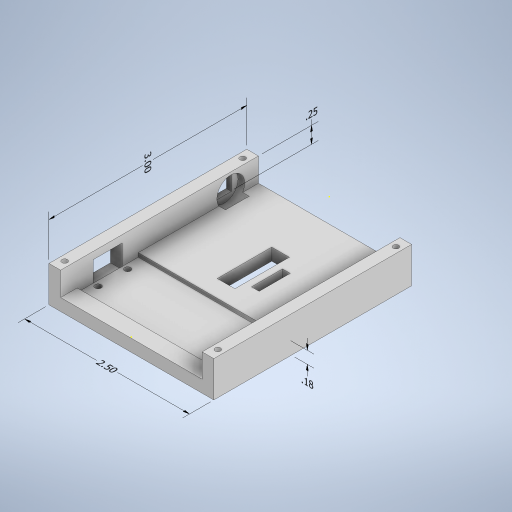
# Autodesk Inventor part: Scanner_Test_Top
Saved by Autodesk Inventor 2024 (Build 280153000, 153)
## iProperties
Created: 2022-09-22
Part Number: Scanner_Test_Top
Material: Generic
Document SubType Name: Modeling
Designer: Vking
Density: 1 g/cm^3
Appearance: Default
Author: Vking
Autodesk Inventor part; units mm, degrees
ref_plane "YZ Plane" through (0, 0, 0) normal (1, 0, 0) x (0, 1, 0)
ref_plane "XZ Plane" through (0, 0, 0) normal (0, 1, 0) x (-1, 0, 0)
ref_plane "XY Plane" through (0, 0, 0) normal (0, 0, 1) x (1, 0, 0)
sketch "Sketch1" plane through (0, 0, 0) normal (0, 0, 1) x (1, 0, 0)
  line L0 (-31.75, 5.08) -> (31.75, 5.08)
  line L1 (31.75, 5.08) -> (31.75, -5.08)
  line L2 (31.75, -5.08) -> (-31.75, -5.08)
  line L3 (-31.75, -5.08) -> (-31.75, 5.08)
  point P0 (0, 0)
  dimension "d0" = 63.5
  dimension "d3" = 31.75
  dimension "d4" = 10.16
  dimension "d17" = 5.08
  constraints: 8 end point, 2 parallel, 1 horizontal, 1 perpendicular
  measures "d0" distance of L0.start L0.end
  measures "d3" distance from line of L3 point (0, 0)
  measures "d4" distance of L0.end L1.end
  measures "d17" distance from line of point (0, 0) L2
extrude "Extrusion1" add sketch "Sketch1" along normal blind 76.2
sketch "Sketch3" plane through (0, 0, 76.2) normal (0, 0, 1) x (1, 0, 0)
  line L0 (-27.25, 0.3875) -> (27.25, 0.3875)
  line L1 (27.25, 0.3875) -> (27.25, -0.3745)
  line L2 (27.25, -0.3745) -> (-27.25, -0.3745)
  line L3 (-27.25, -0.3745) -> (-27.25, 0.3875)
  line L4 (-31.75, 5.08) -> (-31.75, -5.08) projected
  point P0 (0, 0)
  point P1 (-27.25, 0.0065)
  dimension "d6" = 0.762
  dimension "d7" = 54.5
  dimension "d8" = 4.5
  constraints: 8 end point, 2 parallel, 1 horizontal, 1 midpoint, 1 perpendicular
  measures "d6" distance between parallel lines of L2 L0
  measures "d7" distance of L0.start L0.end
  measures "d8" distance from line of L4 point (-27.25, 0.006)
extrude "Extrusion2" cut sketch "Sketch3" against normal blind 85.1
sketch "Sketch8" plane through (0, 0, 76.2) normal (0, 0, 1) x (1, 0, 0)
  line L0 (-31.75, -5.08) -> (31.75, -5.08) projected
  line L1 (31.75, -5.08) -> (31.75, 5.08) projected
  line L2 (-31.75, -5.08) -> (31.75, -5.08)
  line L3 (31.75, -5.08) -> (31.75, 0.3875)
  line L4 (31.75, 0.3875) -> (-31.75, 0.3875)
  line L5 (27.25, 0.3875) -> (27.25, -0.3745) projected
  line L6 (27.25, -0.3745) -> (-27.25, -0.3745) projected
  line L7 (-27.25, -0.3745) -> (-27.25, 0.3875) projected
  line L8 (-27.25, 0.3875) -> (27.25, 0.3875) projected
  line L9 (-31.75, -5.08) -> (31.75, -5.08) projected
  line L10 (31.75, -5.08) -> (31.75, 5.08) projected
  line L11 (31.75, 5.08) -> (-31.75, 5.08) projected
  line L12 (-31.75, 5.08) -> (-31.75, -5.08) projected
  line L13 (-27.25, 0.3875) -> (-27.25, -0.3745) projected
  line L14 (-27.25, 0.3875) -> (27.25, 0.3875)
  line L15 (27.25, 0.3875) -> (27.25, -5.08)
  line L16 (27.25, -5.08) -> (-27.25, -5.08)
  line L17 (-27.25, -5.08) -> (-27.25, 0.3875)
  point P0 (0, 0)
  dimension "d30" = 0
  constraints: 14 end point, 3 parallel, 2 horizontal, 2 perpendicular, 2 point on line
  measures "d30" distance between parallel lines of L8 L4
sketch "Sketch9" plane through (-31.75, 5.08, 0) normal (0, 1, 0) x (1, 0, 0)
  line L0 (28.35, -18.7333) -> (35.15, -18.7333)
  line L1 (35.15, -18.7333) -> (35.15, -39.7333)
  line L2 (35.15, -39.7333) -> (28.35, -39.7333)
  line L3 (28.35, -39.7333) -> (28.35, -18.7333)
  line L4 (0, 0) -> (0, -76.2) projected
  line L5 (63.5, 0) -> (0, 0) projected
  point P0 (31.75, 0)
  point P1 (0, -38.1)
  dimension "d31" = 21
  dimension "d32" = 6.8
  dimension "d33" = 28.35
  dimension "d34" = 18.7333
  constraints: 8 end point, 2 parallel, 1 horizontal, 1 midpoint, 1 perpendicular
  measures "d31" distance of L0.end L1.end
  measures "d32" distance of L1.end L2.end
  measures "d33" distance from line of point (0, -38.1) L3
  measures "d34" distance between parallel lines of L0 L5
extrude "Extrusion6" cut sketch "Sketch8" against normal blind 76.2 contours L17 L6 L15 L0
sketch "Sketch11" plane through (0, 0, 76.2) normal (0, 0, 1) x (1, 0, 0)
  point P0 (0, 0)
sketch "Sketch12" plane through (-31.75, -5.08, 0) normal (0, -1, 0) x (1, 0, 0)
  line L0 (4.5, 0) -> (4.5, 76.2) projected
  line L1 (0, 76.2) -> (4.5, 76.2) projected
  line L2 (0, 0) -> (0, 76.2) projected
  line L3 (0, 0) -> (4.5, 0) projected
  line L4 (59, 76.2) -> (59, 0) projected
  line L5 (59, 0) -> (63.5, 0) projected
  line L6 (63.5, 0) -> (63.5, 76.2) projected
  line L7 (59, 76.2) -> (63.5, 76.2) projected
  point P0 (31.75, 0)
extrude "Extrusion7" add sketch "Sketch12" along normal blind 3.641
extrude "Extrusion8" cut sketch "Sketch9" against normal blind 19.5
sketch "Sketch13" plane through (-31.75, -8.721, 0) normal (0, -1, 0) x (1, 0, 0)
  point P0 (31.75, 0)
sketch "Sketch14" plane through (27.25, 0.3875, 0) normal (-1, 0, 0) x (0, 0, 1)
  circle A0 centre (10.668, -2.7585) radius 5.334
  line L0 (76.2, 0) -> (0, 0) projected
  line L1 (76.2, -9.1085) -> (0, -9.1085) projected
  line L2 (0, -9.1085) -> (0, 0) projected
  point P0 (0, -0.3875)
  dimension "d41" = 10.668
  dimension "d43" = 6.35
  dimension "d44" = 10.668
  constraints: 1 centre point
  measures "d41" diameter of A0
  measures "d43" distance from line of A0.centre L1
  measures "d44" distance from line of A0.centre L2
extrude "Extrusion9" cut sketch "Sketch14" along normal mid plane 5.08
sketch "Sketch17" plane through (-31.75, -8.721, 0) normal (0, -1, 0) x (1, 0, 0)
  circle A0 centre (61.25, 3.81) radius 1.05
  line L0 (59, 0) -> (63.5, 0) projected
  line L1 (59, 76.2) -> (59, 0) projected
  circle A1 centre (2.25, 3.81) radius 1.05
  line L2 (0, 76.2) -> (0, 0) projected
  line L3 (0, 0) -> (4.5, 0) projected
  circle A2 centre (2.25, 72.39) radius 1.05
  circle A3 centre (61.25, 72.39) radius 1.05
  line L4 (4.5, 76.2) -> (0, 76.2) projected
  line L5 (63.5, 76.2) -> (59, 76.2) projected
  point P0 (31.75, 0)
  dimension "d98" = 2.1
  dimension "d99" = 3.81
  dimension "d100" = 2.25
  dimension "d101" = 2.25
  dimension "d102" = 2.1
  dimension "d103" = 3.81
  dimension "d104" = 2.1
  dimension "d105" = 2.1
  dimension "d106" = 3.81
  dimension "d107" = 3.81
  dimension "d108" = 2.25
  constraints: 4 centre point
  measures "d98" diameter of A0
  measures "d99" distance from line of L0 A0.centre
  measures "d100" distance from line of A0.centre L1
  measures "d101" distance from line of L2 A1.centre
  measures "d102" diameter of A1
  measures "d103" distance from line of L3 A1.centre
  measures "d104" diameter of A2
  measures "d105" diameter of A3
  measures "d106" distance from line of A2.centre L4
  measures "d107" distance from line of A3.centre L5
  measures "d108" distance from line of L1 A3.centre
extrude "Extrusion11" cut sketch "Sketch17" against normal blind 5.08
sketch "Sketch20" plane through (-31.75, 5.08, 0) normal (0, 1, 0) x (1, 0, 0)
  line L0 (22.81, -23.9233) -> (25.81, -23.9233)
  line L1 (25.81, -23.9233) -> (25.81, -35.9233)
  line L2 (25.81, -35.9233) -> (22.81, -35.9233)
  line L3 (22.81, -35.9233) -> (22.81, -23.9233)
  line L4 (28.35, -39.7333) -> (28.35, -18.7333) projected
  line L5 (35.15, -39.7333) -> (28.35, -39.7333) projected
  point P0 (31.75, 0)
  point P1 (31.75, -39.7333)
  dimension "d141" = 3
  dimension "d142" = 2.54
  dimension "d143" = 12
  dimension "d144" = 3.81
  constraints: 8 end point, 2 parallel, 1 horizontal, 1 midpoint, 1 perpendicular
  measures "d141" distance between parallel lines of L1 L3
  measures "d142" distance between parallel lines of L4 L1
  measures "d143" distance of L0.end L1.end
  measures "d144" distance from line of point (31.75, -39.733) L2
extrude "Extrusion14" cut sketch "Sketch20" against normal blind 25.4
sketch "Sketch18" plane through (-27.25, 0.3875, 76.2) normal (0, -1, 0) x (1, 0, 0)
  circle A0 centre (5.5, -23.82) radius 1.15
  circle A1 centre (5.5, -12.42) radius 1.05
  circle A2 centre (5.5, -12.42) radius 1.15
  line L0 (3.5, -28.62) -> (3.5, -7.62)
  circle A3 centre (5.5, -23.82) radius 1.05
  line L1 (54.5, -28.62) -> (3.5, -28.62)
  line L2 (3.5, -7.62) -> (54.5, -7.62)
  circle A4 centre (52.5, -12.42) radius 1.05
  circle A5 centre (52.5, -12.42) radius 1.15
  line L3 (54.5, -7.62) -> (54.5, -28.62)
  circle A6 centre (52.5, -23.82) radius 1.05
  circle A7 centre (52.5, -23.82) radius 1.15
  line L4 (0, 0) -> (54.5, 0) projected
  line L5 (54.5, 0) -> (54.5, -76.2) projected
  point P0 (27.25, -76.2)
  dimension "d111" = 21
  dimension "d112" = 51
  dimension "d113" = 2.1
  dimension "d114" = 2.1
  dimension "d115" = 2.1
  dimension "d116" = 2.1
  dimension "d117" = 2
  dimension "d118" = 2
  dimension "d119" = 2
  dimension "d120" = 2
  dimension "d121" = 11.4
  dimension "d122" = 4.8
  dimension "d123" = 11.4
  dimension "d124" = 4.8
  dimension "d125" = 0.1
  dimension "d126" = 0.1
  dimension "d127" = 0.1
  dimension "d128" = 0.1
  dimension "d131" = 7.62
  dimension "d132" = 0
  constraints: 8 centre point, 8 end point, 2 parallel, 1 perpendicular
  measures "d111" distance of L0.start L0.end
  measures "d112" distance of L0.end L2.end
  measures "d113" diameter of A3
  measures "d114" diameter of A1
  measures "d115" diameter of A4
  measures "d116" diameter of A6
  measures "d117" distance from line of A0.centre L0
  measures "d118" distance from line of A1.centre L0
  measures "d119" distance from line of L3 A4.centre
  measures "d120" distance from line of L3 A6.centre
  measures "d121" distance of A1.centre A0.centre
  measures "d122" distance from line of L1 A0.centre
  measures "d123" distance of A4.centre A6.centre
  measures "d124" distance from line of L2 A4.centre
  measures "d125" radial gap between concentric circles of A3 A0
  measures "d126" radial gap between concentric circles of A1 A2
  measures "d127" radial gap between concentric circles of A6 A7
  measures "d128" radial gap between concentric circles of A4 A5
  measures "d131" distance between parallel lines of L4 L2
  measures "d132" distance between parallel lines of L5 L3
extrude "Extrusion12" cut sketch "Sketch18" against normal blind 25.4 contours A0 | A1 | A2 | A3 | A4 | A5 | A6 | A7
sketch "Sketch21" plane through (-31.75, -8.721, 0) normal (0, -1, 0) x (1, 0, 0)
  line L0 (59, 76.2) -> (59, 0) projected
  line L1 (59, 69.5452) -> (61.2521, 69.5452)
  line L2 (61.2521, 69.5452) -> (61.2521, 46.6852)
  line L3 (61.2521, 46.6852) -> (59, 46.6852)
  line L4 (59, 46.6852) -> (59, 69.5452)
  line L5 (63.5, 0) -> (63.5, 76.2) projected
  line L6 (63.5, 76.2) -> (59, 76.2) projected
  point P0 (31.75, 0)
  dimension "d147" = 4.5
  dimension "d148" = 2.2479
  dimension "d149" = 6.6548
  dimension "d150" = 22.86
  constraints: 8 end point, 2 parallel, 1 horizontal, 1 perpendicular, 1 point on line
  measures "d147" distance between parallel lines of L0 L5
  measures "d148" distance between parallel lines of L2 L5
  measures "d149" distance between parallel lines of L6 L1
  measures "d150" distance of L1.end L2.end
sketch "Sketch22" plane through (31.75, 5.08, 76.2) normal (1, 0, 0) x (0, 0, -1)
  line L0 (13.57, -4.6925) -> (13.57, 0) projected
  line L1 (13.57, -4.6925) -> (13.57, 0) projected
  line L2 (24.97, -4.6925) -> (24.97, 0) projected
  line L3 (22.67, -4.6925) -> (22.67, 0) projected
  line L4 (11.27, -4.6925) -> (11.27, 0) projected
  line L5 (23.7, -2.1525) -> (12.54, -2.1525)
  line L6 (12.54, -2.1525) -> (12.54, -11.0425)
  line L7 (12.54, -11.0425) -> (23.7, -11.0425)
  line L8 (23.7, -11.0425) -> (23.7, -2.1525)
  point P0 (76.2, -5.08)
  point P1 (24.97, -2.1525)
  point P2 (11.27, -2.6605)
  dimension "d152" = 8.89
  dimension "d153" = 2.54
  dimension "d169" = 1.27
  dimension "d170" = 1.27
  constraints: 8 end point, 2 parallel, 1 horizontal, 1 perpendicular
  measures "d152" distance of L5.end L6.end
  measures "d153" distance from line of L2.start L5
  measures "d169" distance between parallel lines of L4 L6
  measures "d170" distance between parallel lines of L8 L2
extrude "Extrusion15" cut sketch "Sketch22" against normal blind 4.5212
sketch "Sketch24" plane through (31.75, 5.08, 76.2) normal (1, 0, 0) x (0, 0, -1)
  line L0 (37.6849, -4.6925) -> (33.6849, -4.6925)
  line L1 (33.6849, -4.6925) -> (33.6849, -7.6925)
  line L2 (33.6849, -7.6925) -> (37.6849, -7.6925)
  line L3 (37.6849, -7.6925) -> (37.6849, -4.6925)
  line L4 (0, -4.6925) -> (76.2, -4.6925) projected
  point P0 (76.2, -5.08)
  point P1 (23.7, -4.6925)
  dimension "d163" = 4
  dimension "d164" = 3
  dimension "d165" = 0
  constraints: 8 end point, 2 parallel, 1 horizontal, 1 perpendicular
  measures "d163" distance of L1.end L2.end
  measures "d164" distance of L0.end L1.end
  measures "d165" distance between parallel lines of L4 L0
extrude "Extrusion16" [suppressed]
sketch "Sketch27" plane through (-27.25, 0.3875, 76.2) normal (0, -1, 0) x (1, 0, 0)
  line L0 (54.5, 0) -> (54.5, -76.2) projected
  line L1 (0, 0) -> (0, -76.2) projected
  line L2 (54.5, -29.89) -> (0, -29.89)
  line L3 (0, -29.89) -> (0, -6.35)
  line L4 (0, -6.35) -> (54.5, -6.35)
  line L5 (54.5, -6.35) -> (54.5, -29.89)
  line L6 (54.5, -28.62) -> (3.5, -28.62) projected
  line L7 (3.5, -7.62) -> (54.5, -7.62) projected
  point P0 (27.25, -76.2)
  point P1 (54.5, -6.35)
  point P2 (0, -29.89)
  dimension "d171" = 1.27
  dimension "d172" = 1.27
  constraints: 8 end point, 2 parallel, 2 point on line, 1 horizontal, 1 perpendicular
  measures "d171" distance between parallel lines of L6 L2
  measures "d172" distance between parallel lines of L7 L4
extrude "Extrusion17" cut sketch "Sketch27" against normal blind 1.5
sketch "Sketch28" plane through (29.79, -2.371, 10.668) normal (-1, 0, 0) x (0, 0, 1)
  line L0 (2.794, -2.794) -> (-2.794, -2.794)
  line L1 (-2.794, -2.794) -> (-2.794, 2.794)
  line L2 (-2.794, 2.794) -> (2.794, 2.794)
  line L3 (2.794, 2.794) -> (2.794, -2.794)
  arc A0 (-4.5653, 2.7585) -> (4.5653, 2.7585) centre (0, 0) ccw projected
  point P0 (-10.668, 2.371)
  dimension "d190" = 5.588
  dimension "d191" = 5.588
  dimension "d192" = 2.794
  dimension "d193" = 2.794
  constraints: 8 end point, 2 parallel, 1 horizontal, 1 perpendicular
  measures "d190" distance of L1.end L2.end
  measures "d191" distance of L0.end L1.end
  measures "d192" distance from line of L0 A0.centre
  measures "d193" distance from line of L1 A0.centre
extrude "Extrusion18" cut sketch "Sketch28" against normal blind 7.62
body "Solid1"
